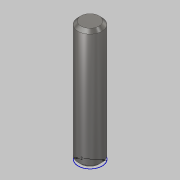
# Autodesk Inventor part: Shaft1
Saved by Autodesk Inventor 2019.2 (Build 232265000, 265)
## iProperties
Created: 2019-01-28
Part Number: Shaft1
Material: Stahl, Legierung
Document SubType Name: Modeling
Designer: Lion
Density: 7.73 g/cm^3
Appearance: Halbpoliert
Mass: 1.21423 g
Surface Area: 3.20442 cm^2
Volume: 0.15708 cm^3
length: 10.000 mm
Author: Lion
Autodesk Inventor part; units mm, degrees
ref_plane "YZ Plane" through (0, 0, 0) normal (1, 0, 0) x (0, 1, 0)
ref_plane "XZ Plane" through (0, 0, 0) normal (0, 1, 0) x (-1, 0, 0)
ref_plane "XY Plane" through (0, 0, 0) normal (0, 0, 1) x (1, 0, 0)
sketch "Skizze1" plane through (0, 0, 0) normal (0, 1, 0) x (-1, 0, 0)
  circle A0 centre (0, 0) radius 1
  dimension "d0" = 2
  constraints: 1 centre point, 1 coincident
  measures "d0" diameter of A0
extrude "Extrusion1" add sketch "Skizze1" along normal blind 10
chamfer "Fase1" distance 0.25 angle 45 2 edges at (1, 10, 0) (1, 0, 0)
